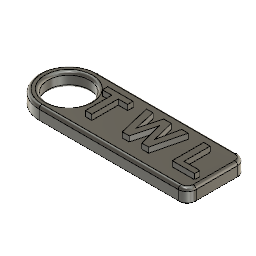
Key Fob v1 (Autodesk Fusion 360 design; units mm, degrees)
Autodesk Fusion 360 part; units mm, degrees
note: some values were not read from the file. Chosen so that the rebuilt part matches the saved one: which bodies a step acts on. Set by a fixed rule: which sketch regions a step uses.
sketch "Sketch1" plane through (0, 0, 0) normal (0, 0, 1) x (1, 0, 0) in component "BASE"
  line L0 (0, 0) -> (50, 0)
  line L1 (50, 0) -> (50, 20)
  line L2 (50, 20) -> (0, 20)
  line L3 (0, 20) -> (0, 0)
  circle A0 centre (0, 10) radius 10
  circle A1 centre (0, 10) radius 7
  dimension "d1" = 50
  dimension "d2" = 20
  dimension "d3" = 14
  measures "d3" diameter of A1
extrude "Extrude1" add sketch "Sketch1" along normal blind 4.8 contours L0 L1 L2 A0 | L3 A0 A1 | L3 A0 A1 makes body 1 in component "BASE"
sketch "Sketch1 (2)" plane through (0, 0, 4.8) normal (0, 0, 1) x (-1, 0, 0) in component "NAME"
  circle A0 centre (0, -10) radius 7
  line L0 (-50, -20) -> (0, -20)
  arc A1 (0, -20) -> (0, 0) centre (0, -10) ccw
  line L1 (0, 0) -> (-50, 0)
  line L2 (-50, 0) -> (-50, -20)
  line L3 (-7.7973, -4.6099) -> (-47.8388, -4.6099) construction
  line L4 (-47.8388, -4.6099) -> (-47.8388, -19.6099) construction
  line L5 (-47.8388, -19.6099) -> (-7.7973, -19.6099) construction
  line L6 (-7.7973, -19.6099) -> (-7.7973, -4.6099) construction
  text T0 "T W L" font "Arial" height 15 bold align ink ink in box 0 x 0 at (-7.8073, -4.6299) x (-1, 0) y (0, -1) spacing 1 height is em
extrude "Extrude1'" add sketch "Sketch1 (2)" along normal blind 1.8 separate body text T0 makes body 2 at (23.0002, 9.3296, 4.8) makes body 3 at (41.0129, 8.7828, 4.8) makes body 4 at (12.4387, 7.6036, 4.8) in component "NAME"
fillet "Fillet1" radius 3 2 edges at (50, 0, 2.4) (50, 20, 2.4) on bodies 1 in component "BASE"
fillet "Fillet2" radius 1 6 edges at (49.1213, 0.8787, 4.8) (50, 10, 4.8) (49.1213, 19.1213, 4.8) (23.5, 20, 4.8) (-10, 10, 4.8) (23.5, 0, 4.8) on bodies 1 in component "BASE"
chamfer "Chamfer1" distance 0.5 angle 45 6 edges at (50, 10, 0) (49.1213, 19.1213, 0) (23.5, 20, 0) (-10, 10, 0) (23.5, 0, 0) (49.1213, 0.8787, 0) on bodies 1 in component "BASE"
fillet "Fillet3" radius 1 2 edges at (-6.5263, 12.5313, 4.8) (-6.5263, 12.5313, 0) on bodies 1 in component "BASE"
component "BASE" placed x (1, 0, 0) y (0, 1, 0) z (0, 0, 1) at (0, 0, 0)
component "NAME" placed x (1, 0, 0) y (0, 1, 0) z (0, 0, 1) at (0, 0, 0)
